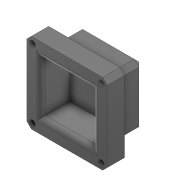
# Autodesk Inventor part: Back cover for servo motor 250 W
Saved by Autodesk Inventor 2020.3 (Build 243373010, 373A)
## iProperties
Created: 2021-04-26
Part Number: Back cover for servo motor 250 W
Material: PBT Plastic
Document SubType Name: Modeling
Designer: marti
Density: 1.31 g/cm^3
Appearance: Smooth - Black
Author: marti
Autodesk Inventor part; units mm, degrees
ref_plane "YZ Plane" through (0, 0, 0) normal (1, 0, 0) x (0, 1, 0)
ref_plane "XZ Plane" through (0, 0, 0) normal (0, 1, 0) x (-1, 0, 0)
ref_plane "XY Plane" through (0, 0, 0) normal (0, 0, 1) x (1, 0, 0)
sketch "Sketch1" plane through (0, 0, 0) normal (0, 0, 1) x (1, 0, 0)
  circle A0 centre (15, -15) radius 1.2295
  circle A1 centre (-15, 15) radius 1.2295
  circle A2 centre (15, 15) radius 1.2295
  circle A3 centre (-15, -15) radius 1.2295
  line L0 (-15.5, -17.5) -> (-17.5, -15.5)
  line L1 (-15.5, -17.5) -> (15.5, -17.5)
  line L2 (17.5, -15.5) -> (15.5, -17.5)
  line L3 (17.5, -15.5) -> (17.5, 15.5)
  line L4 (15.5, 17.5) -> (17.5, 15.5)
  line L5 (15.5, 17.5) -> (-15.5, 17.5)
  line L6 (-17.5, 15.5) -> (-15.5, 17.5)
  line L7 (-17.5, 15.5) -> (-17.5, -15.5)
  point P0 (0, 0)
  point P1 (0, 0)
  point P2 (0, 0)
  constraints: 16 end point, 4 centre point
extrude "Extrusion1" add sketch "Sketch1" along normal mid plane 7.5
sketch "Sketch4" plane through (0, 0, -3.75) normal (0, 0, -1) x (-1, 0, 0)
  line L0 (-13.25, 13.25) -> (13.25, 13.25)
  line L1 (13.25, 13.25) -> (13.25, -13.25)
  line L2 (13.25, -13.25) -> (-13.25, -13.25)
  line L3 (-13.25, -13.25) -> (-13.25, 13.25)
  line L4 (-17.5, 15.5) -> (-17.5, -15.5) projected
  line L5 (15.5, 17.5) -> (-15.5, 17.5) projected
  point P0 (0, 0)
  point P1 (-13.25, 0)
  point P2 (0, 13.25)
  dimension "d15" = 4.25
  dimension "d16" = 4.25
  constraints: 8 end point, 2 midpoint, 2 parallel, 1 horizontal, 1 horizontal alignment, 1 perpendicular, 1 vertical alignment
  measures "d15" distance between parallel lines of L4 L3
  measures "d16" distance between parallel lines of L5 L0
extrude "Extrusion4" add sketch "Sketch4" along normal blind 12.5
sketch "Sketch5" plane through (0, 0, 3.75) normal (0, 0, 1) x (1, 0, 0)
  line L0 (13.25, -13.25) -> (-13.25, -13.25) projected
  line L1 (-13.25, -13.25) -> (-13.25, 13.25) projected
  line L2 (-13.25, 13.25) -> (13.25, 13.25) projected
  line L3 (13.25, 13.25) -> (13.25, -13.25) projected
  line L4 (-11.25, -11.25) -> (11.25, -11.25)
  line L5 (11.25, -11.25) -> (11.25, 11.25)
  line L6 (11.25, 11.25) -> (-11.25, 11.25)
  line L7 (-11.25, 11.25) -> (-11.25, -11.25)
  point P0 (0, 0)
  dimension "d19" = 2
  constraints: 8 end point, 3 other
  measures "d19" distance between parallel lines of L0 L4
extrude "Extrusion5" cut sketch "Sketch5" against normal blind 12.5 contours L7 L6 L5 L4
fillet "Fillet2" radius 2 4 edges at (11.25, 0, 3.75) (-11.25, 0, 3.75) (0, 11.25, 3.75) (0, -11.25, 3.75)
chamfer "Chamfer2" distance 2 angle 45 8 edges at (13.25, -13.25, -10) (13.25, 13.25, -10) (-13.25, -13.25, -10) (-13.25, 13.25, -10) (0, -13.25, -16.25) (13.25, 0, -16.25) (0, 13.25, -16.25) (-13.25, 0, -16.25)
fillet "Fillet3" radius 2 8 edges at (13.25, 0, -3.75) (12.25, 12.25, -3.75) (0, 13.25, -3.75) (-12.25, 12.25, -3.75) (-13.25, 0, -3.75) (-12.25, -12.25, -3.75) (0, -13.25, -3.75) (12.25, -12.25, -3.75)
body "Solid1"
